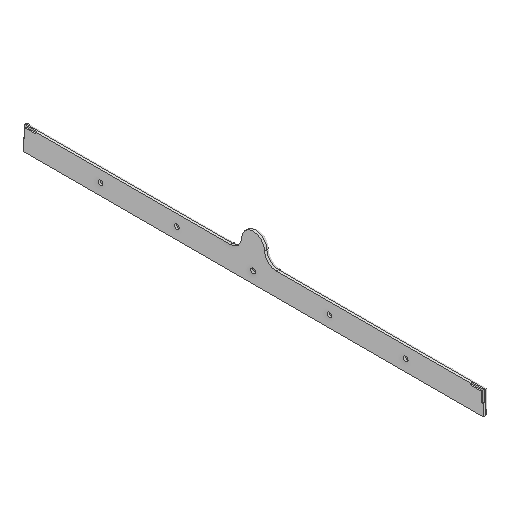
# Autodesk Inventor part: drzalo_za_poster_40x60_top
Saved by Autodesk Inventor 2026 (Build 300175050, 175E)
## iProperties
Created: 2026-05-26
Part Number: drzalo_za_poster_40x60_top
Material: Generic
Document SubType Name: Modeling
Designer: student
Density: 1 g/cm^3
Appearance: Default
Author: student
Autodesk Inventor part; units mm, degrees
ref_plane "YZ Plane" through (0, 0, 0) normal (1, 0, 0) x (0, 1, 0)
ref_plane "XZ Plane" through (0, 0, 0) normal (0, 1, 0) x (-1, 0, 0)
ref_plane "XY Plane" through (0, 0, 0) normal (0, 0, 1) x (1, 0, 0)
sketch "Sketch1" plane through (0, 0, 0) normal (0, 0, 1) x (1, 0, 0)
  line L0 (-200, 10) -> (200, 10)
  line L1 (200, 10) -> (200, -10)
  line L2 (200, -10) -> (-200, -10)
  line L3 (-200, -10) -> (-200, 10)
  circle A0 centre (-133.3333, 0) radius 2.15
  circle A1 centre (-66.6667, 0) radius 2.15
  circle A2 centre (0, 0) radius 2.15
  circle A3 centre (66.6667, 0) radius 2.15
  circle A4 centre (133.3333, 0) radius 2.15
  line L4 (-10, 10) -> (10, 10)
  line L5 (10, 10) -> (10, 30)
  line L6 (10, 30) -> (-10, 30)
  line L7 (-10, 30) -> (-10, 10)
  line L8 (-200, -10) -> (-201, -10)
  line L9 (-201, -10) -> (-201, 10)
  line L10 (-201, 10) -> (-200, 10)
  line L11 (-200, 10) -> (-200, -10)
  line L12 (200, -10) -> (201, -10)
  line L13 (201, -10) -> (201, 10)
  line L14 (201, 10) -> (200, 10)
  line L15 (200, 10) -> (200, -10)
  point P0 (0, 0)
  point P1 (0, 10)
  point P2 (200, 0)
  point P3 (-200, 0)
  point P4 (0, 30)
  dimension "d0" = 400
  dimension "d1" = 20
  dimension "d2" = 4.3
  dimension "d3" = 66.6667
  dimension "d6" = 66.6667
  dimension "d21" = 20
  dimension "d22" = 20
  dimension "d45" = 1
  dimension "d46" = 1
  constraints: 32 end point, 8 parallel, 5 centre point, 5 horizontal, 4 midpoint, 4 perpendicular, 2 horizontal alignment, 2 vertical alignment, 1 point on line, 8 other
  measures "d0" distance of L0.start L0.end
  measures "d1" distance of L0.end L1.end
  measures "d2" diameter of A0
  measures "d3" distance from line of L3 A0.centre
  measures "d6" distance of A0.centre A1.centre
  measures "d21" distance of L4.end L5.end
  measures "d22" distance of L5.end L6.end
  measures "d45" distance of L9.end L10.end
  measures "d46" distance of L14.end L13.end
extrude "Extrusion1" add sketch "Sketch1" along normal blind 5
fillet "Fillet1" radius 10 4 edges at (10, 10, 2.5) (10, 30, 2.5) (-10, 10, 2.5) (-10, 30, 2.5)
extrude "Extrusion2" add sketch "Sketch1" along normal blind 3.2 contours A0 | A1 | A2 | A3 | A4
sketch "Sketch3" plane through (-190, 10, 0) normal (0, 1, 0) x (1, 0, 0)
  line L0 (190, 0) -> (190, -5)
  line L1 (390, -5) -> (210, -5) projected
  circle A0 centre (190, -2.5) radius 2
  line L2 (190.5, -4.5) -> (189.5, -4.5)
  line L3 (189.5, -4.5) -> (189.5, -0.5)
  line L4 (189.5, -0.5) -> (190.5, -0.5)
  line L5 (190.5, -0.5) -> (190.5, -4.5)
  point P0 (380, -5)
  point P1 (0, -5)
  point P2 (190, -4.5)
  point P3 (189.5, -2.5)
  point P4 (190.5, -0.5635)
  point P5 (190.5, -4.4365)
  dimension "d18" = 4
  dimension "d19" = 1
  constraints: 10 end point, 3 midpoint, 2 parallel, 1 centre point, 1 horizontal, 1 horizontal alignment, 1 perpendicular, 1 point on line, 1 tangent, 1 vertical alignment
  measures "d18" diameter of A0
  measures "d19" distance between parallel lines of L5 L3
revolve "Revolution2" [suppressed]
sketch "Sketch4" plane through (0, 0, 0) normal (0, 0, -1) x (-1, 0, 0)
  arc A0 (10, 20) -> (-10, 20) centre (0, 20) ccw projected
  circle A1 centre (0, 20) radius 6
  line L0 (-6, 20) -> (6, 20)
  line L1 (6, 20) -> (6, 5)
  line L2 (6, 5) -> (-6, 5)
  line L3 (-6, 5) -> (-6, 13.2336)
  line L4 (-6, 20) -> (-4, 20)
  line L5 (-4, 20) -> (-4, 17.7057)
  line L6 (-6, 16.9596) -> (-6, 20)
  line L7 (0, 5) -> (0, 6)
  circle A2 centre (0, 11) radius 6
  arc A3 (-5, 15.4697) -> (-4, 17.7057) centre (-7, 17.7057) ccw
  arc A4 (-5, 15.4697) -> (-6, 13.2336) centre (-3, 13.2336) ccw
  line L8 (-6, 13.2336) -> (-6, 16.9596)
  line L9 (4, 20) -> (4, 17.7057)
  arc A5 (4, 17.7057) -> (5, 15.4697) centre (7, 17.7057) ccw
  arc A6 (6, 13.2336) -> (5, 15.4697) centre (3, 13.2336) ccw
  circle A7 centre (0, 20) radius 4
  point P0 (0, 0)
  point P1 (-4, 15)
  point P2 (6, 13.2336)
  point P3 (-6, 18.4798)
  point P4 (4.5061, 16.0383)
  point P5 (-4.5061, 16.0383)
  dimension "d36" = 8
  dimension "d38" = 2
  dimension "d25" = 15
  dimension "d27" = 2.8
  dimension "d28" = 5
  dimension "d30" = 3
  dimension "d39" = 12
  constraints: 20 end point, 9 point on circle, 6 symmetric about line, 5 centre point, 4 tangent, 3 midpoint, 3 parallel, 2 horizontal, 2 perpendicular, 2 point on line, 1 coincident, 1 equal radius, 1 vertical, 1 vertical alignment, 8 other
  measures "d25" distance of L0.end L1.end
  measures "d27" distance of point (-4, 15) L6.start
  measures "d28" distance of L4.end point (-4, 15)
  measures "d30" radius of A3
  measures "d39" diameter of A2
extrude "Extrusion3" [suppressed]
extrude "Extrusion4" add sketch "Sketch4" against normal blind 1 contours L0 A7 A1 | L1 A6 A5 A1 | A1 A5 L9 L0 | L0 L5 A3 A1 | A1 A3 A4 L8 L6
ref_plane "Work Plane1" through (-4, 17.7057, 0) normal (0, -1, 0) x (1, 0, 0)
sketch "Sketch5" plane through (-4, 17.7057, 0) normal (0, -1, 0) x (1, 0, 0)
  line L0 (8, 1) -> (10, 3)
  line L1 (8, 1) -> (10.8284, 1) construction
  line L2 (10, 3) -> (10, 1)
  line L3 (10, 1) -> (8, 1)
  point P0 (4, 0)
  dimension "d40" = 45
  constraints: 8 end point, 1 equal length, 1 horizontal, 1 vertical
  measures "d40" angle of L1 L0
sketch "Sketch6" plane through (0, 0, 0) normal (0, 0, -1) x (-1, 0, 0)
  line L0 (-4, 17.7057) -> (-4, 20) projected
  arc A0 (4, 20) -> (-4, 20) centre (0, 20) ccw projected
  line L1 (4, 20) -> (4, 17.7057) projected
  point P0 (0, 0)
sweep "Sweep1" [suppressed]
fillet "Fillet2" [suppressed]
fillet "Fillet3" radius 3 5 edges at (-10, 20, 0) (10, 20, 0) (7.0712, 27.0712, 0) (201, 0, 0) (-201, 0, 0)
sketch "Sketch7" plane through (0, 0, 5) normal (0, 0, 1) x (1, 0, 0)
  line L0 (-20, 10) -> (-201, 10) projected
  line L1 (-201, 10) -> (-200, 10)
  line L2 (-200, 10) -> (-200, 0)
  line L3 (-200, 0) -> (-201, 0)
  line L4 (-201, 0) -> (-201, 10)
  line L5 (-200, 10) -> (-190, 10)
  line L6 (-190, 10) -> (-190, 9)
  line L7 (-190, 9) -> (-200, 9)
  line L8 (-200, 9) -> (-200, 10)
  line L9 (0, 0) -> (0, 1.5374)
  line L10 (20, 10) -> (201, 10)
  line L11 (201, 10) -> (200, 10)
  line L12 (200, 10) -> (200, 0)
  line L13 (200, 0) -> (201, 0)
  line L14 (201, 0) -> (201, 10)
  line L15 (200, 10) -> (190, 10)
  line L16 (190, 10) -> (190, 9)
  line L17 (190, 9) -> (200, 9)
  line L18 (200, 9) -> (200, 10)
  line L19 (-200, 0) -> (-199.6, 0)
  line L20 (-199.6, 0) -> (-199.6, 9)
  line L21 (-199.6, 9) -> (-200, 9)
  line L22 (-200, 9) -> (-200, 0)
  line L23 (-190, 9) -> (-200, 9)
  line L24 (-200, 9) -> (-200, 8.6)
  line L25 (-200, 8.6) -> (-190, 8.6)
  line L26 (-190, 8.6) -> (-190, 9)
  line L27 (190, 9) -> (200, 9)
  line L28 (200, 9) -> (200, 8.6)
  line L29 (200, 8.6) -> (190, 8.6)
  line L30 (190, 8.6) -> (190, 9)
  line L31 (200, 0) -> (199.6, 0)
  line L32 (199.6, 0) -> (199.6, 8.6)
  line L33 (199.6, 8.6) -> (200, 8.6)
  line L34 (200, 8.6) -> (200, 0)
  point P0 (-199.6, 8.6)
  dimension "d47" = 1
  dimension "d48" = 10
  dimension "d49" = 10
  dimension "d50" = 1
  dimension "d53" = 0.4
  dimension "d54" = 0.4
  dimension "d55" = 0.4
  dimension "d56" = 0.4
  constraints: 68 end point, 12 parallel, 8 symmetric about line, 6 horizontal, 6 perpendicular, 4 point on line, 1 vertical
  measures "d47" distance of L2.end L3.end
  measures "d48" distance of L1.end L2.end
  measures "d49" distance of L6.end L7.end
  measures "d50" distance of L5.end L6.end
  measures "d53" distance of L21.end L20.end
  measures "d54" distance of L24.end L23.end
  measures "d55" distance of L27.end L28.end
  measures "d56" distance of L32.end L33.end
extrude "Extrusion5" cut sketch "Sketch7" against normal blind 1
equation "\"d0\" = dolzina_drzala"
equation "\"d1\" = sirina_drzala"
equation "\"d2\" = fi_magneta + 2 * toleranca"
equation "\"d6\" = d3"
equation "\"d11\" = debelina_drzala"
equation "\"d14\" = -globina_luknje + debelina_drzala - toleranca"
equation "\"d27\" = -0.5 * d23 + 0.5 * d24"
equation "\"d39\" = d36 + 2 * d38"
equation "\"fi_magneta\" = 3.7"
equation "\"toleranca\" = 0.3"
equation "\"dolzina_drzala\" = 400"
equation "\"sirina_drzala\" = 20"
equation "\"debelina_drzala\" = 5"
equation "\"globina_luknje\" = 1.5"
equation "\"d23\" = 4.4"
equation "\"d24\" = 10"
body "Solid1"
